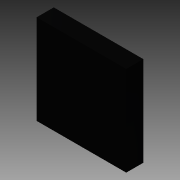
# Autodesk Inventor part: TMP006
Saved by Autodesk Inventor 2013 (Build 170138000, 138)
## iProperties
Created: 2015-06-30
Part Number: TMP006
Material: Ogólny
Document SubType Name: Modeling
Designer: terg
Density: 1 g/cm^3
Author: terg
Autodesk Inventor part; units mm, degrees
ref_plane "YZ Plane" through (0, 0, 0) normal (1, 0, 0) x (0, 1, 0)
ref_plane "XZ Plane" through (0, 0, 0) normal (0, 1, 0) x (-1, 0, 0)
ref_plane "XY Plane" through (0, 0, 0) normal (0, 0, 1) x (1, 0, 0)
sketch "Szkic1" plane through (0, 0, 0) normal (0, 1, 0) x (-1, 0, 0)
  line L0 (0, 0) -> (1.565, 0)
  line L1 (1.565, 0) -> (1.565, 1.565)
  line L2 (1.565, 1.565) -> (0, 1.565)
  line L3 (0, 1.565) -> (0, 0)
  dimension "d0" = 1.565
  dimension "d1" = 1.565
  constraints: 8 end point, 2 parallel, 1 horizontal, 1 perpendicular
  measures "d0" distance of L2.end L1.end
  measures "d1" distance of L1.end L0.end
extrude "Wyciągnięcie proste1" add sketch "Szkic1" along normal blind 0.3
sketch "Szkic2" plane through (0, 0.3, 0) normal (0, 1, 0) x (1, 0, 0)
  line L0 (-1.565, 0) -> (-1.265, 0)
  line L1 (-1.265, 0) -> (-1.265, -0.3)
  line L2 (-1.265, -0.3) -> (-1.565, -0.3)
  line L3 (-1.565, -0.3) -> (-1.565, 0)
  dimension "d4" = 0.3
  dimension "d5" = 0.3
  constraints: 8 end point, 2 parallel, 1 horizontal, 1 perpendicular
  measures "d4" distance of L1.end L2.end
  measures "d5" distance of L0.end L1.end
extrude "Wyciągnięcie proste2" cut sketch "Szkic2" against normal blind 0.03
